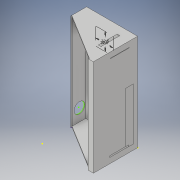
# Autodesk Inventor part: caixa interruptors
Saved by Autodesk Inventor 2019 (Build 230136000, 136)
## iProperties
Created: 2018-08-12
Part Number: caixa interruptors
Material: Genérico
Document SubType Name: Modeling
Designer: Albert Garangou Culebras
Density: 1 g/cm^3
Appearance: Valor por defecto
Author: Albert Garangou Culebras
Autodesk Inventor part; units mm, degrees
ref_plane "YZ Plane" through (0, 0, 0) normal (1, 0, 0) x (0, 1, 0)
ref_plane "XZ Plane" through (0, 0, 0) normal (0, 1, 0) x (-1, 0, 0)
ref_plane "XY Plane" through (0, 0, 0) normal (0, 0, 1) x (1, 0, 0)
sketch "Boceto15" plane through (0, 0, 0) normal (0, 1, 0) x (-1, 0, 0)
  line L0 (0, 0) -> (0, -82.5)
  line L1 (0, -82.5) -> (95.1, -82.5)
  line L2 (0, 0) -> (10, 0)
  line L3 (8.9499, -1.7021) -> (94.0499, -54.2021)
  line L4 (8.9499, -1.7021) -> (8.7796, -1.5971)
  line L5 (8.7796, -1.5971) -> (9.7649, 0)
  line L6 (10, 0) -> (9.7649, 0)
  line L7 (94.0499, -54.2021) -> (94.2201, -54.3072)
  line L8 (94.2201, -54.3072) -> (95.1, -52.8809)
  line L9 (95.1, -52.8809) -> (95.1, -82.5)
  dimension "d61" = 2
  dimension "d62" = 0.2
  constraints: 20 end point, 3 perpendicular, 2 vertical, 1 collinear, 1 horizontal, 1 point on line
  measures "d61" distance of L2.end L3.start
  measures "d62" distance of L3.end L7.end
extrude "Extrusión15" add sketch "Boceto15" along normal blind 180
sketch "Boceto16" plane through (0, 0, 0) normal (0, -1, 0) x (1, 0, 0)
  line L0 (-95.1, -52.8809) -> (-94.2201, -54.3072) projected
  line L1 (-94.2201, -54.3072) -> (-94.2201, -79.5002)
  line L2 (0, -82.5) -> (-95.1, -82.5) projected
  line L3 (-94.2201, -79.5002) -> (-2.0001, -79.5002)
  line L4 (0, 0) -> (0, -82.5) projected
  line L5 (-2.0001, -79.5002) -> (-2.0001, -1.7331)
  line L6 (-2.0001, -1.7331) -> (-9, -1.7331)
  line L7 (-94.2201, -54.3072) -> (-8.7796, -1.5971) projected
  line L8 (-94.2201, -54.3072) -> (-8.7796, -1.5971)
  dimension "d65" = 25.193
  dimension "d66" = 92.22
  constraints: 10 end point, 2 perpendicular, 2 point on line, 1 collinear, 1 horizontal, 1 parallel
  measures "d65" distance of L0.end L1.end
  measures "d66" distance of L1.end L3.end
extrude "Extrusión16" cut sketch "Boceto16" against normal blind 178
sketch "Boceto17" plane through (0, 0, 0) normal (0, -1, 0) x (1, 0, 0)
  line L0 (-9, -1.7331) -> (-2.0001, -1.7331) projected
  line L1 (-94.2201, -54.3072) -> (-9, -1.7331) projected
  line L2 (-9, -1.7331) -> (-94.2201, -54.3072)
  line L3 (-2.0001, -79.5002) -> (-94.2201, -79.5002) projected
  line L4 (-94.2201, -54.3072) -> (-94.2201, -79.5002)
  line L5 (-94.2201, -79.5002) -> (-2.0001, -79.5002)
  line L6 (-2.0001, -1.7331) -> (-2.0001, -79.5002) projected
  line L7 (-2.0001, -79.5002) -> (-2.0001, -1.7331)
  line L8 (-2.0001, -1.7331) -> (-9, -1.7331)
  point P0 (0, 0)
  constraints: 10 end point, 3 perpendicular, 2 collinear
extrude "Extrusión17" add sketch "Boceto17" against normal blind 2
sketch "Boceto18" plane through (-95.1, 0, -82.5) normal (-1, 0, 0) x (0, 0, 1)
  line L0 (0, 0) -> (29.6191, 0) projected
  line L1 (0, 0) -> (29.6191, 0)
  circle A0 centre (14.8095, 25) radius 10
  point P0 (82.5, 0)
  constraints: 2 end point, 1 centre point, 1 collinear
extrude "Extrusión18" cut sketch "Boceto18" against normal blind 17.5
sketch "Boceto23" plane through (0, 0, -82.5) normal (0, 0, -1) x (-1, 0, 0)
  line L0 (0, 0) -> (0, 180) projected
  line L1 (0, 180) -> (0, 160)
  line L2 (81, 160) -> (76, 160)
  line L3 (76, 160) -> (76, 155)
  line L4 (76, 155) -> (81, 155)
  line L5 (81, 155) -> (81, 160)
  line L6 (46, 160) -> (48, 160)
  line L7 (48, 160) -> (48, 155)
  line L8 (48, 155) -> (43, 155)
  line L9 (43, 155) -> (43, 160)
  line L10 (43, 160) -> (48, 160)
  line L11 (46, 127) -> (48, 127)
  line L12 (48, 127) -> (48, 122)
  line L13 (48, 122) -> (43, 122)
  line L14 (43, 127) -> (43, 122)
  line L15 (43, 127) -> (46, 127)
  line L16 (81, 125) -> (81, 127)
  line L17 (81, 127) -> (76, 127)
  line L18 (76, 124) -> (76, 127)
  line L19 (81, 122) -> (81, 125)
  line L20 (81, 155) -> (81, 127)
  line L21 (76, 160) -> (48, 160)
  line L22 (76, 124) -> (76, 122)
  line L23 (76, 122) -> (81, 122)
  line L24 (48, 122) -> (76, 122)
  line L25 (43, 127) -> (43, 155)
  dimension "d119" = 20
  constraints: 50 end point, 5 perpendicular, 5 vertical, 3 collinear, 3 horizontal, 2 parallel
  measures "d119" distance of L1.end L0.end
sketch "Boceto24" plane through (0, 0, -82.5) normal (0, 0, -1) x (-1, 0, 0)
  circle A0 centre (78.3646, 157.5) radius 1.5
  circle A1 centre (78.3646, 124.5) radius 1.5
  circle A2 centre (45.3646, 124.5) radius 1.5
  circle A3 centre (45.3646, 157.5) radius 1.5
  line L0 (43.3646, 157.5) -> (45.3646, 157.5)
  line L1 (43.3646, 122.5) -> (43.3646, 124.5)
  line L2 (78.3646, 122.5) -> (78.3646, 124.5)
  line L3 (43.3646, 124.5) -> (45.3646, 124.5)
  point P0 (0, 0)
  dimension "d129" = 3
  dimension "d181" = 2
  dimension "d182" = 2
  dimension "d183" = 2
  dimension "d184" = 2
  constraints: 8 end point, 4 centre point, 2 horizontal, 2 vertical
  measures "d129" diameter of A3
  measures "d181" distance of L0.start L0.end
  measures "d182" distance of L1.start L1.end
  measures "d183" distance of L2.start L2.end
  measures "d184" distance of L1.end L3.end
extrude "Extrusión24" cut sketch "Boceto24" against normal blind 10
sketch "Boceto25" plane through (0, 0, -82.5) normal (0, 0, -1) x (-1, 0, 0)
  line L0 (0, 0) -> (0, 180) projected
  line L1 (95.1, 0) -> (95.1, 180) projected
  line L2 (0, 0) -> (95.1, 0) projected
  line L3 (21.275, 42.5) -> (21.275, 12.5)
  line L4 (21.275, 42.5) -> (21.275, 72.5)
  line L5 (26.275, 72.5) -> (26.275, 12.5)
  line L6 (26.275, 12.5) -> (21.275, 12.5)
  line L7 (45.05, 72.5) -> (45.05, 12.5)
  line L8 (45.05, 12.5) -> (50.05, 12.5)
  line L9 (50.05, 12.5) -> (50.05, 72.5)
  line L10 (68.825, 72.5) -> (68.825, 12.5)
  line L11 (68.825, 12.5) -> (73.825, 12.5)
  line L12 (73.825, 12.5) -> (73.825, 63)
  line L13 (73.825, 63) -> (73.825, 72.5)
  line L14 (73.825, 72.5) -> (73.825, 85)
  line L15 (68.825, 85) -> (68.825, 72.5)
  line L16 (50.05, 72.5) -> (50.05, 85)
  line L17 (45.05, 85) -> (45.05, 72.5)
  line L18 (26.275, 72.5) -> (26.275, 85)
  line L19 (21.275, 85) -> (21.275, 72.5)
  line L20 (73.825, 85) -> (73.825, 95)
  line L21 (73.825, 95) -> (68.825, 95)
  line L22 (68.825, 95) -> (68.825, 85)
  line L23 (50.05, 85) -> (50.05, 95)
  line L24 (50.05, 95) -> (45.05, 95)
  line L25 (45.05, 95) -> (45.05, 85)
  line L26 (26.275, 85) -> (26.275, 95)
  line L27 (26.275, 95) -> (21.275, 95)
  line L28 (21.275, 95) -> (21.275, 85)
  dimension "d134" = 30
  dimension "d135" = 30
  dimension "d136" = 5
  dimension "d138" = 5
  dimension "d140" = 5
  dimension "d146" = 10
  constraints: 52 end point, 8 perpendicular, 4 vertical, 1 point on line
  measures "d134" distance of L3.start L3.end
  measures "d135" distance of L3.start L4.end
  measures "d136" distance of L4.end L5.start
  measures "d138" distance of L7.end L8.end
  measures "d140" distance of L10.end L11.end
  measures "d146" distance of L14.end L20.end
sketch "Boceto26" plane through (0, 0, 0) normal (0, -1, 0) x (1, 0, 0)
  line L0 (0, -82.5) -> (-95.1, -82.5) projected
  line L1 (-57, -82.5) -> (-29, -66.3342)
  line L2 (-57, -82.5) -> (-24.6684, -82.5) construction
  point P0 (0, 0)
  dimension "d141" = 30
  constraints: 4 end point, 1 equal length, 1 horizontal, 1 point on line
  measures "d141" angle of L2 L1
sweep "Barrido1" cut profiles "Boceto25" path "Boceto26" path curves L1
sketch "Boceto27" plane through (-2.0001, 178, -79.5002) normal (-1, 0, 0) x (0, 0, 1)
  line L0 (5, -101) -> (5, -167)
  line L1 (5, -167) -> (16, -167)
  line L2 (19, -168) -> (5, -168)
  line L3 (5, -168) -> (5, -71)
  line L4 (5, -71) -> (19, -71)
  line L5 (19, -71) -> (19, -168)
  point P0 (79.5002, -178)
  constraints: 12 end point, 2 parallel, 1 horizontal, 1 perpendicular, 1 point on line
extrude "Extrusión25" add sketch "Boceto27" against normal blind 2.0002
sketch "Boceto28" plane through (0, 0, 0) normal (0, -1, 0) x (1, 0, 0)
  line L0 (0, -82.5) -> (-95.1, -82.5) projected
  line L1 (0, -82.5) -> (-20, -82.5)
  line L2 (-20, -82.5) -> (-20, -9)
  line L3 (-17.5, -45.75) -> (-17.5, -65.75)
  line L4 (-17.5, -65.75) -> (-22.5, -65.75)
  line L5 (-22.5, -65.75) -> (-22.5, -45.75)
  line L6 (-22.5, -45.75) -> (-22.5, -30.75)
  line L7 (-22.5, -30.75) -> (-17.5, -30.75)
  line L8 (-17.5, -30.75) -> (-17.5, -45.75)
  point P0 (0, 0)
  dimension "d147" = 20
  dimension "d149" = 20
  dimension "d150" = 5
  dimension "d151" = 20
  dimension "d153" = 5
  constraints: 16 end point, 3 perpendicular, 3 point on line
  measures "d147" distance of L0.start L1.end
  measures "d149" distance of L3.start L3.end
  measures "d150" distance of L3.end L4.end
  measures "d151" distance of L4.end L5.end
  measures "d153" distance of L6.end L7.end
sketch "Boceto29" plane through (0, 180, 0) normal (0, 1, 0) x (1, 0, 0)
  line L0 (0, 82.5) -> (-95.1, 82.5) projected
  line L1 (0, 82.5) -> (-20, 82.5)
  line L2 (-20, 82.5) -> (-20, 11)
  line L3 (-20, 46.75) -> (-17.5, 46.75)
  line L4 (-17.5, 46.75) -> (-17.5, 31.75)
  line L5 (-17.5, 31.75) -> (-22.5, 31.75)
  line L6 (-22.5, 31.75) -> (-22.5, 46.75)
  line L7 (-22.5, 46.75) -> (-22.5, 66.75)
  line L8 (-22.5, 66.75) -> (-17.5, 66.75)
  line L9 (-17.5, 66.75) -> (-17.5, 46.75)
  point P0 (0, 0)
  dimension "d154" = 20
  dimension "d155" = 2.5
  dimension "d156" = 15
  dimension "d157" = 5
  dimension "d158" = 15
  dimension "d159" = 20
  dimension "d160" = 5
  constraints: 18 end point, 4 perpendicular, 4 point on line, 1 horizontal, 1 midpoint
  measures "d154" distance of L0.start L1.end
  measures "d155" distance of L3.start L3.end
  measures "d156" distance of L3.end L4.end
  measures "d157" distance of L4.end L5.end
  measures "d158" distance of L5.end L6.end
  measures "d159" distance of L6.end L7.end
  measures "d160" distance of L7.end L8.end
sketch "Boceto30" plane through (0, 0, -82.5) normal (0, 0, -1) x (-1, 0, 0)
  line L0 (0, 180) -> (95.1, 180) projected
  line L1 (25, 180) -> (6, 169.0303)
  line L2 (25, 180) -> (46.9393, 180) construction
  point P0 (0, 0)
  dimension "d161" = 150
  constraints: 4 end point, 1 equal length, 1 horizontal, 1 point on line
  measures "d161" angle of L1 L2
sweep "Barrido2" cut profiles "Boceto29" path "Boceto30" path curves L1
sketch "Boceto31" plane through (0, 0, -82.5) normal (0, 0, -1) x (-1, 0, 0)
  line L0 (40, 0) -> (17, 13.2791)
  line L1 (40, 0) -> (66.5581, 0) construction
  point P0 (0, 0)
  dimension "d164" = 150
  constraints: 4 end point, 1 equal length, 1 horizontal
  measures "d164" angle of L1 L0
sweep "Barrido3" cut profiles "Boceto28" path "Boceto31"
sketch "Boceto32" plane through (-2.0001, 178, -79.5002) normal (-1, 0, 0) x (0, 0, 1)
  line L0 (9, -172) -> (54, -172)
  line L1 (54, -172) -> (54, -161)
  line L2 (54, -161) -> (9, -161)
  line L3 (9, -161) -> (9, -172)
  line L4 (9, -15) -> (51, -15)
  line L5 (51, -15) -> (51, -3)
  line L6 (51, -3) -> (9, -3)
  line L7 (9, -3) -> (9, -15)
  point P0 (79.5002, -178)
  constraints: 16 end point, 4 parallel, 2 horizontal, 2 perpendicular, 1 point on line
extrude "Extrusión26" add sketch "Boceto32" against normal blind 2
sketch "Boceto33" plane through (0, 0, -82.5) normal (0, 0, -1) x (-1, 0, 0)
  line L0 (2, 160) -> (17, 160)
  line L1 (17, 160) -> (17, 120)
  line L2 (17, 120) -> (2, 120)
  line L3 (2, 120) -> (2, 160)
  point P0 (0, 0)
  constraints: 8 end point, 2 parallel, 1 horizontal, 1 perpendicular
extrude "Extrusión27" cut sketch "Boceto33" against normal blind 4
sketch "Boceto34" plane through (-94.2201, 178, -54.3072) normal (1, 0, 0) x (0, 0, -1)
  line L0 (0, -176) -> (25.193, -176) projected
  line L1 (0, -176) -> (0, 0) projected
  line L2 (25.193, -176) -> (0, -176)
  line L3 (0, -176) -> (0, 0)
  line L4 (0, 0) -> (25.193, 0)
  line L5 (25.193, 0) -> (25.193, -176)
  point P0 (-54.3072, -178)
  constraints: 8 end point, 2 parallel, 1 horizontal, 1 perpendicular
extrude "Extrusión28" add sketch "Boceto34" along normal blind 0.5
sketch "Boceto36" plane through (0, 2, 0) normal (0, 1, 0) x (1, 0, 0)
  line L0 (-94.2201, 54.3072) -> (-9, 1.7331) projected
  line L1 (-93.7201, 54.3072) -> (-94.2201, 54.3072) projected
  line L2 (-94.2201, 54.3072) -> (-93.7201, 54.3072)
  line L3 (-94.2201, 54.3072) -> (-93.6573, 53.9599)
  line L4 (-93.7201, 54.3072) -> (-93.858, 54.0837)
  point P0 (0, 0)
  constraints: 6 end point, 2 point on line, 1 collinear, 1 perpendicular
extrude "Extrusión29" add sketch "Boceto36" along normal blind 178
sketch "Boceto37" plane through (0, 0, -82.5) normal (0, 0, -1) x (-1, 0, 0)
  circle A0 centre (78.3646, 157.5) radius 1.5 projected
  line L0 (78.3646, 157.5) -> (78.3646, 125)
  line L1 (78.3646, 157.5) -> (45.8646, 157.5)
  point P0 (0, 0)
  dimension "d175" = 32.5
  dimension "d177" = 32.5
  constraints: 4 end point, 1 horizontal, 1 vertical
  measures "d175" distance of L0.start L0.end
  measures "d177" distance of L0.start L1.end
extrude "Extrusión30" cut sketch "Boceto23" against normal blind 178 contours L3 L4 L20 L17 L18 L22 L24 L12 L11 L15 L25 L8 L7 L21
extrude "Extrusión31" cut sketch "Boceto18" against normal blind 53.25
